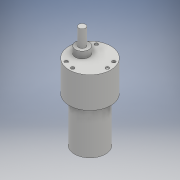
# Autodesk Inventor part: 380-300c1
Saved by Autodesk Inventor 2018 (Build 220112000, 112)
## iProperties
Created: 2018-11-27
Part Number: 380-300c1
Material: 一般
Document SubType Name: Modeling
Designer: shun2
Density: 1 g/cm^3
Appearance: 既定
Author: shun2
Autodesk Inventor part; units mm, degrees
ref_plane "YZ Plane" through (0, 0, 0) normal (1, 0, 0) x (0, 1, 0)
ref_plane "XZ Plane" through (0, 0, 0) normal (0, 1, 0) x (-1, 0, 0)
ref_plane "XY Plane" through (0, 0, 0) normal (0, 0, 1) x (1, 0, 0)
sketch "スケッチ1" plane through (0, 0, 0) normal (0, 0, 1) x (1, 0, 0)
  circle A0 centre (0, 0) radius 13.75
  dimension "d0" = 27.5
  constraints: 1 centre point, 1 coincident
  measures "d0" diameter of A0
extrude "押し出し1" add sketch "スケッチ1" along normal blind 38
sketch "スケッチ2" plane through (0, 0, 38) normal (0, 0, 1) x (1, 0, 0)
  circle A0 centre (0, 0) radius 15
  dimension "d3" = 30
  constraints: 1 centre point, 1 coincident
  measures "d3" diameter of A0
extrude "押し出し2" add sketch "スケッチ2" along normal blind 2
sketch "スケッチ3" plane through (0, 0, 40) normal (0, 0, 1) x (1, 0, 0)
  circle A0 centre (0, 0) radius 18.5
  dimension "d6" = 37
  constraints: 1 centre point, 1 coincident
  measures "d6" diameter of A0
extrude "押し出し3" add sketch "スケッチ3" along normal blind 27.5
sketch "スケッチ4" plane through (0, 0, 0) normal (0, 0, -1) x (-1, 0, 0)
  circle A0 centre (0, 0) radius 5.1
  dimension "d9" = 10.2
  constraints: 1 centre point, 1 coincident
  measures "d9" diameter of A0
extrude "押し出し4" add sketch "スケッチ4" along normal blind 3
sketch "スケッチ5" plane through (0, 0, 67.5) normal (0, 0, 1) x (1, 0, 0)
  circle A0 centre (-7, 0) radius 6
  point P0 (0, 0)
  dimension "d12" = 12
  constraints: 1 centre point, 1 coincident
  measures "d12" diameter of A0
extrude "押し出し5" add sketch "スケッチ5" along normal blind 6
sketch "スケッチ6" plane through (-7, 0, 73.5) normal (0, 0, 1) x (1, 0, 0)
  circle A0 centre (0, 0) radius 3
  point P0 (7, 0)
  dimension "d15" = 6
  constraints: 1 centre point
  measures "d15" diameter of A0
extrude "押し出し6" add sketch "スケッチ6" along normal blind 15
sketch "スケッチ7" plane through (0, 0, 67.5) normal (0, 0, 1) x (1, 0, 0)
  circle A0 centre (-7.75, -13.4234) radius 1.5
  circle A1 centre (-7.75, 13.4234) radius 1.5
  circle A2 centre (15.5, 0) radius 1.5
  circle A3 centre (0, -15.5) radius 1.5
  circle A4 centre (-13.4234, 7.75) radius 1.5
  circle A5 centre (13.4234, 7.75) radius 1.5
  point P0 (0, 0)
  point P1 (0, 0)
  point P2 (0, 0)
  dimension "d19" = 3
  dimension "d20" = 3
  dimension "d21" = 3
  dimension "d22" = 3
  dimension "d23" = 3
  dimension "d24" = 3
  constraints: 6 centre point, 1 coincident
  measures "d19" diameter of A0
  measures "d20" diameter of A1
  measures "d21" diameter of A2
  measures "d22" diameter of A3
  measures "d23" diameter of A4
  measures "d24" diameter of A5
extrude "押し出し7" cut sketch "スケッチ7" against normal blind 15 contours A3 | A4 | A5
sketch "スケッチ8" plane through (0, 0, 67.5) normal (0, 0, 1) x (1, 0, 0)
  circle A0 centre (-7.75, -13.4234) radius 1.5
  circle A1 centre (-7.75, 13.4234) radius 1.5
  circle A2 centre (15.5, 0) radius 1.5
  circle A3 centre (0, -15.5) radius 1.5
  circle A4 centre (-13.4234, 7.75) radius 1.5
  circle A5 centre (13.4234, 7.75) radius 1.5
  point P0 (0, 0)
  point P1 (0, 0)
  point P2 (0, 0)
  point P3 (0, 0)
  dimension "d27" = 3
  dimension "d28" = 3
  dimension "d29" = 3
  dimension "d30" = 3
  dimension "d31" = 3
  dimension "d32" = 3
  constraints: 6 centre point, 1 coincident
  measures "d27" diameter of A0
  measures "d28" diameter of A1
  measures "d29" diameter of A2
  measures "d30" diameter of A3
  measures "d31" diameter of A4
  measures "d32" diameter of A5
extrude "押し出し8" cut sketch "スケッチ8" against normal blind 1 contours A0 | A1 | A2
